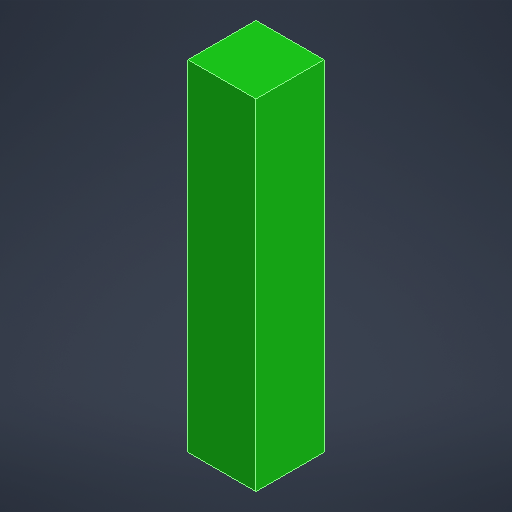
# Autodesk Inventor part: Pieza3
Saved by Autodesk Inventor 2026 (Build 300175050, 175E)
## iProperties
Created: 2025-06-14
Part Number: Pieza3
Material: MDF Tablero de fibras de densidad media
Document SubType Name: Modeling
Designer: renato
Density: 0.8 g/cm^3
Appearance: Verde oscuro
Mass: 0.628319 g
Surface Area: 4.71239 cm^2
Volume: 0.785398 cm^3
Author: renato
Autodesk Inventor part; units mm, degrees
ref_plane "YZ Plane" through (0, 0, 0) normal (1, 0, 0) x (0, 1, 0)
ref_plane "XZ Plane" through (0, 0, 0) normal (0, 1, 0) x (-1, 0, 0)
ref_plane "XY Plane" through (0, 0, 0) normal (0, 0, 1) x (1, 0, 0)
sketch "Boceto2" plane through (0, 0, 0) normal (0, 0, 1) x (1, 0, 0)
  line L0 (-5, -25) -> (5, -25)
  line L1 (5, -25) -> (5, 25)
  line L2 (5, 25) -> (-5, 25)
  line L3 (-5, 25) -> (-5, -25)
  line L4 (-5, -25) -> (5, 25) construction
  line L5 (5, -25) -> (-5, 25) construction
  point P0 (0, 0)
  dimension "d3" = 10
  dimension "d4" = 50
  constraints: 12 end point, 2 midpoint, 2 parallel, 1 horizontal, 1 perpendicular
  measures "d3" distance of L2.end L1.end
  measures "d4" distance of L1.end L0.end
extrude "Extrusión2" add sketch "Boceto2" along normal blind 10
